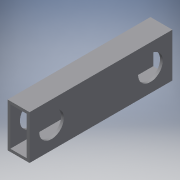
# Autodesk Inventor part: intake srms
Saved by Autodesk Inventor 2018.2 (Build 222227000, 227)
## iProperties
Created: 2018-02-01
Part Number: intake srms
Material: Generic
Document SubType Name: Modeling
Designer: jahu2
Density: 1 g/cm^3
Appearance: Default
Author: jahu2
Autodesk Inventor part; units mm, degrees
ref_plane "YZ Plane" through (0, 0, 0) normal (1, 0, 0) x (0, 1, 0)
ref_plane "XZ Plane" through (0, 0, 0) normal (0, 1, 0) x (-1, 0, 0)
ref_plane "XY Plane" through (0, 0, 0) normal (0, 0, 1) x (1, 0, 0)
sketch "Sketch1" plane through (0, 0, 0) normal (0, 0, 1) x (1, 0, 0)
  line L0 (0, 0) -> (-25.4, 0)
  line L1 (-25.4, 0) -> (-25.4, -50.8)
  line L2 (-25.4, -50.8) -> (0, -50.8)
  line L3 (0, -50.8) -> (0, 0)
  line L4 (-22.225, -3.175) -> (-3.175, -3.175)
  line L5 (-3.175, -3.175) -> (-3.175, -47.625)
  line L6 (-3.175, -47.625) -> (-22.225, -47.625)
  line L7 (-22.225, -47.625) -> (-22.225, -3.175)
  dimension "d0" = 25.4
  dimension "d1" = 50.8
  dimension "d2" = 3.175
  constraints: 16 end point, 4 parallel, 2 perpendicular, 1 horizontal, 3 other
  measures "d0" distance of L2.end L1.end
  measures "d1" distance of L1.end L0.end
  measures "d2" distance between parallel lines of L0 L4
extrude "Extrusion1" add sketch "Sketch1" along normal blind 165.1
sketch "Sketch2" plane through (0, -50.8, 0) normal (1, 0, 0) x (0, 0, -1)
  circle A0 centre (-25.4, 25.4) radius 14.2875
  line L0 (0, 0) -> (0, 50.8) projected
  line L1 (0, 50.8) -> (-165.1, 50.8) projected
  circle A1 centre (-139.7, 25.4) radius 14.2875
  line L2 (0, 0) -> (-165.1, 0) projected
  line L3 (-165.1, 0) -> (-165.1, 50.8) projected
  dimension "d5" = 28.575
  dimension "d6" = 25.4
  dimension "d7" = 25.4
  dimension "d8" = 28.575
  dimension "d9" = 25.4
  dimension "d10" = 25.4
  constraints: 2 centre point
  measures "d5" diameter of A0
  measures "d6" distance from line of L0 A0.centre
  measures "d7" distance from line of L1 A0.centre
  measures "d8" diameter of A1
  measures "d9" distance from line of L2 A1.centre
  measures "d10" distance from line of L3 A1.centre
extrude "Extrusion2" cut sketch "Sketch2" against normal blind 177.8 contours A0 | A1
body "Solid1"
